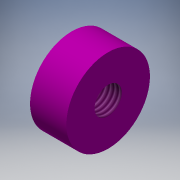
# Autodesk Inventor part: Roller End Plug
Saved by Autodesk Inventor 2017 (Build 210142000, 142)
## iProperties
Created: 2017-01-14
Part Number: Roller End Plug
Material: Generic
Document SubType Name: Modeling
Designer: Ben
Density: 1 g/cm^3
Appearance: Magenta
Author: Ben
Autodesk Inventor part; units mm, degrees
ref_plane "YZ Plane" through (0, 0, 0) normal (1, 0, 0) x (0, 1, 0)
ref_plane "XZ Plane" through (0, 0, 0) normal (0, 1, 0) x (-1, 0, 0)
ref_plane "XY Plane" through (0, 0, 0) normal (0, 0, 1) x (1, 0, 0)
sketch "Sketch3" plane through (0, 0, 0) normal (1, 0, 0) x (0, 1, 0)
  circle A0 centre (0, 0) radius 15.875 construction
  circle A1 centre (0, 0) radius 14.6304
  circle A2 centre (0, 0) radius 4.7625
  dimension "d8" = 31.75
  dimension "d9" = 1.2446
  dimension "d15" = 9.525
  dimension "d22" = 29.2608
  constraints: 3 centre point, 3 coincident
  measures "d8" diameter of A0
  measures "d9" radial gap between concentric circles of A0 A1
  measures "d15" diameter of A2
  measures "d22" diameter of A1
extrude "Extrusion3" add sketch "Sketch3" along normal blind 12.7
thread "Thread1" size "3/8-16 UNC" class "2B" standard "ANSI Unified Screw Threads" full length
body "Solid2"
